Autodesk Fusion 360 part; units mm, degrees
(part 9 of 21)
  spline S252 degree 3 poles (-27.9507, 7.0582) (-27.9377, 7.0577) (-27.9248, 7.0598) (-27.9003, 7.0688) (-27.8891, 7.0756) (-27.8724, 7.0909) (-27.8662, 7.0984) (-27.8563, 7.115) (-27.8526, 7.124) (-27.8502, 7.1333) knots 0 0 0 0 0.003906 0.003906 0.007813 0.007813 0.010709 0.010709 0.013605 0.013605 0.013605 0.013605
  spline S253 degree 5 poles (-27.9507, 7.0582) (-27.9531, 7.0583) (-27.9637, 7.0587) (-27.9826, 7.0593) (-28.0098, 7.0601) (-28.0453, 7.061) (-28.0868, 7.0618) (-28.1283, 7.0622) (-28.1698, 7.0625) (-28.2114, 7.0625) (-28.253, 7.0622) (-28.2947, 7.0618) (-28.3364, 7.0611) (-28.3781, 7.0601) (-28.4199, 7.059) (-28.4617, 7.0576) (-28.5036, 7.0559) (-28.5454, 7.0541) (-28.5873, 7.0521) (-28.6293, 7.0498) (-28.6712, 7.0474) (-28.7132, 7.0447) (-28.7553, 7.0419) (-28.7973, 7.0388) (-28.8394, 7.0356) (-28.8815, 7.0321) (-28.9236, 7.0285) (-28.9658, 7.0247) (-29.0079, 7.0207) (-29.0501, 7.0165) (-29.0923, 7.0121) (-29.1346, 7.0075) (-29.1768, 7.0027) (-29.2191, 6.9978) (-29.2614, 6.9927) (-29.3037, 6.9874) (-29.3461, 6.982) (-29.3884, 6.9763) (-29.4308, 6.9705) (-29.4732, 6.9646) (-29.5156, 6.9584) (-29.558, 6.9521) (-29.6004, 6.9456) (-29.6429, 6.939) (-29.6854, 6.9321) (-29.7278, 6.9252) (-29.7703, 6.918) (-29.8128, 6.9107) (-29.8553, 6.9033) (-29.8979, 6.8956) (-29.9404, 6.8879) (-29.983, 6.8799) (-30.0255, 6.8718) (-30.0681, 6.8636) (-30.1107, 6.8552) (-30.1533, 6.8466) (-30.1873, 6.8396) (-30.2129, 6.8343) (-30.2299, 6.8308) (-30.2385, 6.829) knots 0.224488 0.224488 0.224488 0.224488 0.224488 0.224488 0.228571 0.242857 0.257143 0.271429 0.285714 0.3 0.314286 0.328571 0.342857 0.357143 0.371429 0.385714 0.4 0.414286 0.428571 0.442857 0.457143 0.471429 0.485714 0.5 0.514286 0.528571 0.542857 0.557143 0.571429 0.585714 0.6 0.614286 0.628571 0.642857 0.657143 0.671429 0.685714 0.7 0.714286 0.728571 0.742857 0.757143 0.771429 0.785714 0.8 0.814286 0.828571 0.842857 0.857143 0.871429 0.885714 0.9 0.914286 0.928571 0.942857 0.957143 0.971429 0.985714 1 1 1 1 1 1
  arc A157 (-30.2385, 6.829) -> (-30.4018, 6.0605) centre (0, 0) ccw
  spline S254 degree 5 poles (-30.4018, 6.0605) (-30.3948, 6.0554) (-30.3806, 6.0452) (-30.3594, 6.03) (-30.3311, 6.0097) (-30.2957, 5.9846) (-30.2602, 5.9596) (-30.2247, 5.9348) (-30.1891, 5.91) (-30.1535, 5.8855) (-30.1178, 5.8611) (-30.082, 5.8368) (-30.0462, 5.8127) (-30.0104, 5.7887) (-29.9744, 5.7649) (-29.9385, 5.7413) (-29.9025, 5.7178) (-29.8664, 5.6945) (-29.8303, 5.6713) (-29.7941, 5.6483) (-29.7578, 5.6254) (-29.7215, 5.6027) (-29.6852, 5.5802) (-29.6488, 5.5578) (-29.6123, 5.5356) (-29.5758, 5.5135) (-29.5393, 5.4917) (-29.5026, 5.47) (-29.466, 5.4484) (-29.4292, 5.4271) (-29.3925, 5.4059) (-29.3556, 5.3849) (-29.3187, 5.3641) (-29.2818, 5.3434) (-29.2448, 5.323) (-29.2077, 5.3027) (-29.1706, 5.2826) (-29.1334, 5.2627) (-29.0962, 5.243) (-29.0589, 5.2235) (-29.0216, 5.2042) (-28.9842, 5.1851) (-28.9467, 5.1662) (-28.9092, 5.1475) (-28.8716, 5.129) (-28.834, 5.1107) (-28.7963, 5.0927) (-28.7586, 5.0749) (-28.7208, 5.0572) (-28.6829, 5.0399) (-28.645, 5.0227) (-28.607, 5.0058) (-28.5689, 4.9891) (-28.5308, 4.9727) (-28.4926, 4.9565) (-28.4599, 4.9429) (-28.4347, 4.9326) (-28.4172, 4.9255) (-28.4073, 4.9215) (-28.4051, 4.9206) knots -1 -1 -1 -1 -1 -1 -0.985714 -0.971429 -0.957143 -0.942857 -0.928571 -0.914286 -0.9 -0.885714 -0.871429 -0.857143 -0.842857 -0.828571 -0.814286 -0.8 -0.785714 -0.771429 -0.757143 -0.742857 -0.728571 -0.714286 -0.7 -0.685714 -0.671429 -0.657143 -0.642857 -0.628571 -0.614286 -0.6 -0.585714 -0.571429 -0.557143 -0.542857 -0.528571 -0.514286 -0.5 -0.485714 -0.471429 -0.457143 -0.442857 -0.428571 -0.414286 -0.4 -0.385714 -0.371429 -0.357143 -0.342857 -0.328571 -0.314286 -0.3 -0.285714 -0.271429 -0.257143 -0.242857 -0.228571 -0.224488 -0.224488 -0.224488 -0.224488 -0.224488 -0.224488
  spline S255 degree 3 poles (-28.3438, 4.8111) (-28.3416, 4.8239) (-28.342, 4.8371) (-28.3477, 4.8625) (-28.353, 4.8745) (-28.366, 4.8931) (-28.3726, 4.9001) (-28.3878, 4.9121) (-28.3961, 4.917) (-28.4051, 4.9206) knots 0 0 0 0 0.003906 0.003906 0.007813 0.007813 0.010709 0.010709 0.013605 0.013605 0.013605 0.013605
  arc A158 (-28.3438, 4.8111) -> (-28.4432, 4.1831) centre (0, 0) ccw
  spline S256 degree 3 poles (-28.5354, 4.0979) (-28.5224, 4.0988) (-28.5097, 4.1022) (-28.4864, 4.1137) (-28.4759, 4.1216) (-28.4609, 4.1386) (-28.4556, 4.1467) (-28.4474, 4.1642) (-28.4447, 4.1735) (-28.4432, 4.1831) knots 0 0 0 0 0.003906 0.003906 0.007813 0.007813 0.010709 0.010709 0.013605 0.013605 0.013605 0.013605
  spline S257 degree 5 poles (-28.5354, 4.0979) (-28.5378, 4.0977) (-28.5484, 4.097) (-28.5672, 4.0957) (-28.5944, 4.0936) (-28.6298, 4.0908) (-28.6711, 4.0872) (-28.7124, 4.0833) (-28.7537, 4.0792) (-28.7951, 4.0749) (-28.8365, 4.0703) (-28.8778, 4.0655) (-28.9192, 4.0604) (-28.9607, 4.0551) (-29.0021, 4.0496) (-29.0435, 4.0438) (-29.085, 4.0379) (-29.1264, 4.0317) (-29.1679, 4.0253) (-29.2094, 4.0186) (-29.2508, 4.0118) (-29.2923, 4.0048) (-29.3338, 3.9976) (-29.3753, 3.9901) (-29.4168, 3.9825) (-29.4583, 3.9747) (-29.4998, 3.9667) (-29.5414, 3.9584) (-29.5829, 3.95) (-29.6244, 3.9415) (-29.6659, 3.9327) (-29.7075, 3.9237) (-29.749, 3.9146) (-29.7905, 3.9053) (-29.8321, 3.8958) (-29.8736, 3.8861) (-29.9151, 3.8762) (-29.9567, 3.8662) (-29.9982, 3.856) (-30.0397, 3.8456) (-30.0812, 3.8351) (-30.1228, 3.8244) (-30.1643, 3.8135) (-30.2058, 3.8024) (-30.2473, 3.7912) (-30.2889, 3.7798) (-30.3304, 3.7683) (-30.3719, 3.7566) (-30.4134, 3.7447) (-30.4549, 3.7327) (-30.4964, 3.7205) (-30.5379, 3.7082) (-30.5793, 3.6957) (-30.6208, 3.683) (-30.6623, 3.6702) (-30.7037, 3.6572) (-30.7369, 3.6467) (-30.7618, 3.6388) (-30.7784, 3.6335) (-30.7866, 3.6308) knots 0.224488 0.224488 0.224488 0.224488 0.224488 0.224488 0.228571 0.242857 0.257143 0.271429 0.285714 0.3 0.314286 0.328571 0.342857 0.357143 0.371429 0.385714 0.4 0.414286 0.428571 0.442857 0.457143 0.471429 0.485714 0.5 0.514286 0.528571 0.542857 0.557143 0.571429 0.585714 0.6 0.614286 0.628571 0.642857 0.657143 0.671429 0.685714 0.7 0.714286 0.728571 0.742857 0.757143 0.771429 0.785714 0.8 0.814286 0.828571 0.842857 0.857143 0.871429 0.885714 0.9 0.914286 0.928571 0.942857 0.957143 0.971429 0.985714 1 1 1 1 1 1
  arc A159 (-30.7866, 3.6308) -> (-30.8688, 2.8495) centre (0, 0) ccw
  spline S258 degree 5 poles (-30.8688, 2.8495) (-30.8612, 2.8451) (-30.8461, 2.8365) (-30.8234, 2.8235) (-30.7932, 2.8064) (-30.7553, 2.7851) (-30.7174, 2.7639) (-30.6795, 2.7429) (-30.6415, 2.722) (-30.6035, 2.7013) (-30.5654, 2.6808) (-30.5273, 2.6604) (-30.4892, 2.6402) (-30.451, 2.6201) (-30.4128, 2.6002) (-30.3746, 2.5804) (-30.3363, 2.5608) (-30.298, 2.5414) (-30.2596, 2.5221) (-30.2213, 2.503) (-30.1828, 2.484) (-30.1444, 2.4653) (-30.1059, 2.4466) (-30.0673, 2.4282) (-30.0287, 2.4099) (-29.9901, 2.3918) (-29.9515, 2.3739) (-29.9128, 2.3561) (-29.8741, 2.3386) (-29.8353, 2.3212) (-29.7965, 2.3039) (-29.7577, 2.2869) (-29.7188, 2.2701) (-29.6799, 2.2534) (-29.641, 2.2369) (-29.602, 2.2206) (-29.563, 2.2045) (-29.5239, 2.1886) (-29.4849, 2.1729) (-29.4457, 2.1574) (-29.4066, 2.1421) (-29.3674, 2.127) (-29.3282, 2.1122) (-29.2889, 2.0975) (-29.2496, 2.083) (-29.2103, 2.0688) (-29.1709, 2.0548) (-29.1315, 2.041) (-29.0921, 2.0274) (-29.0526, 2.0141) (-29.0131, 2.001) (-28.9735, 1.9881) (-28.9339, 1.9755) (-28.8943, 1.9632) (-28.8546, 1.9511) (-28.8206, 1.9409) (-28.7945, 1.9333) (-28.7763, 1.9281) (-28.7661, 1.9252) (-28.7638, 1.9245) knots -1 -1 -1 -1 -1 -1 -0.985714 -0.971429 -0.957143 -0.942857 -0.928571 -0.914286 -0.9 -0.885714 -0.871429 -0.857143 -0.842857 -0.828571 -0.814286 -0.8 -0.785714 -0.771429 -0.757143 -0.742857 -0.728571 -0.714286 -0.7 -0.685714 -0.671429 -0.657143 -0.642857 -0.628571 -0.614286 -0.6 -0.585714 -0.571429 -0.557143 -0.542857 -0.528571 -0.514286 -0.5 -0.485714 -0.471429 -0.457143 -0.442857 -0.428571 -0.414286 -0.4 -0.385714 -0.371429 -0.357143 -0.342857 -0.328571 -0.314286 -0.3 -0.285714 -0.271429 -0.257143 -0.242857 -0.228571 -0.224488 -0.224488 -0.224488 -0.224488 -0.224488 -0.224488
  spline S259 degree 3 poles (-28.6914, 1.822) (-28.6906, 1.835) (-28.6923, 1.848) (-28.7006, 1.8727) (-28.7072, 1.8841) (-28.7221, 1.9012) (-28.7294, 1.9075) (-28.7457, 1.9179) (-28.7546, 1.9219) (-28.7638, 1.9245) knots 0 0 0 0 0.003906 0.003906 0.007813 0.007813 0.010709 0.010709 0.013605 0.013605 0.013605 0.013605
  line L20 (0, 31) -> (0, 3.7492)
  line L21 (2.2037, 3.0332) -> (18.2213, 25.0795)
  circle A160 centre (0, 0) radius 7.5
  circle A161 centre (0, 0) radius 27.5
  dimension "d19" = 36
  dimension "d20" = 15
  dimension "d21" = 55
  constraint vertical L20
  constraint coincident A1.centre L20
  constraint coincident A1.centre L21
  constraint coincident A9 L20.end
  constraint coincident A13 L21.start
  constraint coincident A131 L20.start
  constraint coincident A119 L21.end
  constraint coincident A1.centre A3.centre
  constraint concentric A1 A161
  measures "d19" angle of L20 L21
  measures "d20" diameter of A160
  measures "d21" diameter of A161
extrude "Estrusione4" cut sketch "Schizzo1 (3)" against normal blind 1 contours L20 L21 A160 A161 picked at (8.9949, 18.7465) bodies 1 in component "Spur Gear (60 teeth)"
pattern_circular "Serie C2" count 5 over 360 about axis through (0, 0, 0) along (0, 0, 1) of "Estrusione4" in component "Spur Gear (60 teeth)"
extrude "Estrusione5" cut 1 faces at (-3.6482, -2.3787, 8) along direction (0, 0, -1) blind 1.6 on bodies 1 bodies 1 in component "Spur Gear (60 teeth)"
sketch "Schizzo2 (3)" plane through (0, 0, 2) normal (0, 0, 1) x (-1, 0, 0)
  line L0 (7.1329, -2.3176) -> (26.1541, -8.498)
  arc A0 (26.1541, -8.498) -> (26.1541, 8.498) centre (0, 0) ccw
  line L1 (26.1541, 8.498) -> (7.1329, 2.3176)
  arc A1 (7.1329, -2.3176) -> (7.1329, 2.3176) centre (0, 0) ccw
  line L2 (24.4009, 8.0452) -> (-1.5991, 8.0452) construction
  line L3 (-1.5991, 8.0452) -> (-1.5991, -2.9548) construction
  line L4 (-1.5991, -2.9548) -> (24.4009, -2.9548) construction
  line L5 (24.4009, -2.9548) -> (24.4009, 8.0452) construction
  dimension "d28" = 5
  text T0 "60s" font "Arial" height 5 bold align left top in box 26 x 11 at (24.4009, 8.0452) x (-1, 0) y (0, -1) spacing 1 kerned
extrude "Estrusione6" add sketch "Schizzo2 (3)" along normal blind 1 text T0 bodies 1 in component "Spur Gear (60 teeth)"
component "Spur Gear (60 teeth)" placed x (1, 0, 0) y (0, 1, 0) z (0, 0, 1) at (0, 0, 0)
component "Spur Gear (10 teeth)" placed x (1, 0, 0) y (0, 1, 0) z (0, 0, 1) at (0, 0, 0)
equation "d19 = ( 360 / 10 ) * 1 deg"

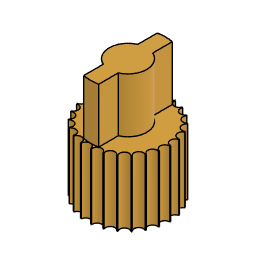
design "2 pomello lancetta secondi"
Autodesk Fusion 360 part; units mm, degrees
sketch "Schizzo1" plane through (0, 0, 0) normal (0, 0, 1) x (1, 0, 0)
  line L0 (0, -45) -> (5, 0)
  line L1 (5, 0) -> (0, 15)
  line L2 (0, 15) -> (-5, 0)
  line L3 (-5, 0) -> (0, -45)
  line L4 (0, -45) -> (0, 15) construction
  line L5 (5, 0) -> (-5, 0) construction
  line L6 (-1, 15) -> (1, 15)
  line L7 (1, 15) -> (1, -45)
  line L8 (1, -45) -> (-1, -45)
  line L9 (-1, -45) -> (-1, 15)
  circle A0 centre (0, 0) radius 5
  dimension "d1" = 45
  dimension "d2" = 15
  dimension "d3" = 5
  dimension "d12" = 1
  dimension "d13" = 1
  constraint vertical L4
  constraint perpendicular L4 L5
  constraint midpoint A0.centre L5
  constraint equal L0 L3
  constraint equal L1 L2
  constraint horizontal L6
  constraint vertical L7
  constraint horizontal L8
  constraint vertical L9
  constraint coincident A0.centre origin
  constraint coincident L0.end A0
  constraint midpoint L0.start L8
  constraint midpoint L1.end L6
  measures "d1" vertical distance of L0.start L0.end
  measures "d2" vertical distance of L0.end L1.end
  measures "d3" horizontal distance of L0.start L0.end
  measures "d12" distance of A0.centre L9
  measures "d13" distance of A0.centre L7
extrude "Estrusione1" add sketch "Schizzo1" along normal blind 2 contours L0 L3 L7 L9 A0 | L3 L8 L9 | L0 L7 L8 | L0 L1 L7 A0 | L0 A0 | L7 L9 A0 | L3 A0 | L2 L3 L9 A0 | L1 A0 | L1 L2 L7 L9 A0 | L2 A0 | L1 L6 L7 | L2 L6 L9
sketch "Schizzo2" plane through (0, 0, 2) normal (0, 0, 1) x (-1, 0, 0)
  circle A0 centre (0, 0) radius 2
  circle A1 centre (0, 0) radius 4
  line L0 (-0.8, 24) -> (0.8, 24)
  line L1 (0.8, 24) -> (0.8, -21)
  line L2 (0.8, -21) -> (-0.8, -21)
  line L3 (-0.8, -21) -> (-0.8, 24)
  arc A2 (-1, 4.899) -> (-1, -4.899) centre (0, 0) ccw
  line L4 (-1, -4.899) -> (-1, -15)
  line L5 (-1, -15) -> (1, -15)
  line L6 (1, -15) -> (1, -4.899)
  arc A3 (1, -4.899) -> (1, 4.899) centre (0, 0) ccw
  line L7 (1, 4.899) -> (1, 45)
  line L8 (-1, 45) -> (-1, 4.899)
  line L9 (1, 45) -> (-1, 45)
  dimension "d6" = 4
  dimension "d7" = 8
  dimension "d8" = 0.8
  dimension "d9" = 0.8
  constraint coincident A0.centre A1.centre
  constraint horizontal L0
  constraint vertical L1
  constraint horizontal L2
  constraint vertical L3
  measures "d6" diameter of A0
  measures "d7" diameter of A1
  measures "d8" distance of A0.centre L3
  measures "d9" distance of A0.centre L1
extrude "Estrusione2" add sketch "Schizzo2" along normal blind 3.8 contours A0 L1 | A0 L1 L3 | A0 A1 L1 L3 | A0 A1 L1 L3 | A0 L3
extrude "Estrusione3" add 1 faces at (0.3333, -45, 0.6667) along direction (0, -1, 0) blind 10
sketch "Schizzo3" plane through (0, 0, 0) normal (0, 0, -1) x (1, 0, 0)
  line L0 (1, 4.899) -> (1, 55)
  line L1 (1, 55) -> (-1, 55)
  line L2 (-1, 55) -> (-1, 4.899)
  arc A0 (-1, 4.899) -> (-1, -4.899) centre (0, 0) ccw
  line L3 (-1, -4.899) -> (-1, -15)
  line L4 (-1, -15) -> (1, -15)
  line L5 (1, -15) -> (1, -4.899)
  arc A1 (1, -4.899) -> (1, 4.899) centre (0, 0) ccw
  circle A2 centre (0, 0) radius 6
  dimension "d16" = 12
  constraint concentric A0 A2
  measures "d16" diameter of A2
extrude "Estrusione4" add sketch "Schizzo3" against normal up to surface (2 mm away) contours L0 L5 A1 A2 | L2 A0 L3 A2
sketch "Schizzo4" plane through (0, 0, 0) normal (0, 0, -1) x (1, 0, 0)
  line L0 (1, 5.9161) -> (1, 55)
  line L1 (1, 55) -> (-1, 55)
  line L2 (-1, 55) -> (-1, 5.9161)
  arc A0 (-1, 5.9161) -> (-1, -5.9161) centre (0, 0) ccw
  line L3 (-1, -5.9161) -> (-1, -15)
  line L4 (-1, -15) -> (1, -15)
  line L5 (1, -15) -> (1, -5.9161)
  arc A1 (1, -5.9161) -> (1, 5.9161) centre (0, 0) ccw
  circle A2 centre (0, 0) radius 4.5
  circle A3 centre (0, 4.5) radius 0.5
  circle A4 centre (-1.0769, 4.3692) radius 0.5
  circle A5 centre (-2.0913, 3.9846) radius 0.5
  circle A6 centre (-2.9841, 3.3683) radius 0.5
  circle A7 centre (-3.7034, 2.5563) radius 0.5
  circle A8 centre (-4.2076, 1.5957) radius 0.5
  circle A9 centre (-4.4672, 0.5424) radius 0.5
  circle A10 centre (-4.4672, -0.5424) radius 0.5
  circle A11 centre (-4.2076, -1.5957) radius 0.5
  circle A12 centre (-3.7034, -2.5563) radius 0.5
  circle A13 centre (-2.9841, -3.3683) radius 0.5
  circle A14 centre (-2.0913, -3.9846) radius 0.5
  circle A15 centre (-1.0769, -4.3692) radius 0.5
  circle A16 centre (0, -4.5) radius 0.5
  circle A17 centre (1.0769, -4.3692) radius 0.5
  circle A18 centre (2.0913, -3.9846) radius 0.5
  circle A19 centre (2.9841, -3.3683) radius 0.5
  circle A20 centre (3.7034, -2.5563) radius 0.5
  circle A21 centre (4.2076, -1.5957) radius 0.5
  circle A22 centre (4.4672, -0.5424) radius 0.5
  circle A23 centre (4.4672, 0.5424) radius 0.5
  circle A24 centre (4.2076, 1.5957) radius 0.5
  circle A25 centre (3.7034, 2.5563) radius 0.5
  circle A26 centre (2.9841, 3.3683) radius 0.5
  circle A27 centre (2.0913, 3.9846) radius 0.5
  circle A28 centre (1.0769, 4.3692) radius 0.5
  dimension "d19" = 9
  dimension "d20" = 1
  dimension "d22" = 360
  constraint coincident A0.centre A1.centre
  constraint coincident A2 A3.centre
  measures "d19" diameter of A2
  measures "d20" diameter of A3
extrude "Estrusione5" add sketch "Schizzo4" along normal blind 7 contours A2 A3 A4 A5 A6 A7 A8 A9 A10 A11 A12 A13 A14 A15 A16 A17 A18 A19 A20 A21 A22 A23 A24 A25 A26 A27 A28
sketch "Schizzo5" plane through (0, 0, 2) normal (0, 0, 1) x (-1, 0, 0)
  line L0 (-0.8, 1.833) -> (-0.8, 3.9192)
  arc A0 (0.8, 3.9192) -> (-0.8, 3.9192) centre (0, 0) ccw
  line L1 (0.8, 3.9192) -> (0.8, 1.833)
  arc A1 (0.8, -1.833) -> (0.8, 1.833) centre (0, 0) ccw
  line L2 (0.8, -1.833) -> (0.8, -3.9192)
  arc A2 (-0.8, -3.9192) -> (0.8, -3.9192) centre (0, 0) ccw
  line L3 (-0.8, -3.9192) -> (-0.8, -1.833)
  arc A3 (-0.8, 1.833) -> (-0.8, -1.833) centre (0, 0) ccw
  line L4 (-1, -5.9161) -> (-1, -15)
  line L5 (-1, -15) -> (1, -15)
  line L6 (1, -15) -> (1, -5.9161)
  arc A4 (1, -5.9161) -> (1, 5.9161) centre (0, 0) ccw
  line L7 (1, 5.9161) -> (1, 55)
  line L8 (1, 55) -> (-1, 55)
  line L9 (-1, 55) -> (-1, 5.9161)
  arc A5 (-1, 5.9161) -> (-1, -5.9161) centre (0, 0) ccw
extrude "Estrusione6" cut sketch "Schizzo5" against normal up to surface (2 mm away)
sketch "Schizzo6" plane through (0, 0, -7) normal (0, 0, -1) x (1, 0, 0)
  arc A0 (2.592, 3.6786) -> (2.5204, 3.728) centre (0, 0) ccw
  arc A1 (1.6363, 4.192) -> (2.5204, 3.728) centre (2.0913, 3.9846) ccw
  arc A2 (1.6363, 4.192) -> (1.555, 4.2228) centre (0, 0) ccw
  arc A3 (0.5856, 4.4617) -> (1.555, 4.2228) centre (1.0769, 4.3692) ccw
  arc A4 (0.5856, 4.4617) -> (0.4992, 4.4722) centre (0, 0) ccw
  arc A5 (-0.4992, 4.4722) -> (0.4992, 4.4722) centre (0, 4.5) ccw
  arc A6 (-0.4992, 4.4722) -> (-0.5856, 4.4617) centre (0, 0) ccw
  arc A7 (-1.555, 4.2228) -> (-0.5856, 4.4617) centre (-1.0769, 4.3692) ccw
  arc A8 (-1.555, 4.2228) -> (-1.6363, 4.192) centre (0, 0) ccw
  arc A9 (-2.5204, 3.728) -> (-1.6363, 4.192) centre (-2.0913, 3.9846) ccw
  arc A10 (-2.5204, 3.728) -> (-2.592, 3.6786) centre (0, 0) ccw
  arc A11 (-3.3393, 3.0165) -> (-2.592, 3.6786) centre (-2.9841, 3.3683) ccw
  arc A12 (-3.3393, 3.0165) -> (-3.397, 2.9514) centre (0, 0) ccw
  arc A13 (-3.9642, 2.1297) -> (-3.397, 2.9514) centre (-3.7034, 2.5563) ccw
  arc A14 (-3.9642, 2.1297) -> (-4.0046, 2.0527) centre (0, 0) ccw
  arc A15 (-4.3586, 1.1191) -> (-4.0046, 2.0527) centre (-4.2076, 1.5957) ccw
  arc A16 (-4.3586, 1.1191) -> (-4.3794, 1.0347) centre (0, 0) ccw
  arc A17 (-4.4998, 0.0435) -> (-4.3794, 1.0347) centre (-4.4672, 0.5424) ccw
  arc A18 (-4.4998, 0.0435) -> (-4.4998, -0.0435) centre (0, 0) ccw
  arc A19 (-4.3794, -1.0347) -> (-4.4998, -0.0435) centre (-4.4672, -0.5424) ccw
  arc A20 (-4.3794, -1.0347) -> (-4.3586, -1.1191) centre (0, 0) ccw
  arc A21 (-4.0046, -2.0527) -> (-4.3586, -1.1191) centre (-4.2076, -1.5957) ccw
  arc A22 (-4.0046, -2.0527) -> (-3.9642, -2.1297) centre (0, 0) ccw
  arc A23 (-3.397, -2.9514) -> (-3.9642, -2.1297) centre (-3.7034, -2.5563) ccw
  arc A24 (-3.397, -2.9514) -> (-3.3393, -3.0165) centre (0, 0) ccw
  arc A25 (-2.592, -3.6786) -> (-3.3393, -3.0165) centre (-2.9841, -3.3683) ccw
  arc A26 (-2.592, -3.6786) -> (-2.5204, -3.728) centre (0, 0) ccw
  arc A27 (-1.6363, -4.192) -> (-2.5204, -3.728) centre (-2.0913, -3.9846) ccw
  arc A28 (-1.6363, -4.192) -> (-1.555, -4.2228) centre (0, 0) ccw
  arc A29 (-0.5856, -4.4617) -> (-1.555, -4.2228) centre (-1.0769, -4.3692) ccw
  arc A30 (-0.5856, -4.4617) -> (-0.4992, -4.4722) centre (0, 0) ccw
  arc A31 (0.4992, -4.4722) -> (-0.4992, -4.4722) centre (0, -4.5) ccw
  arc A32 (0.4992, -4.4722) -> (0.5856, -4.4617) centre (0, 0) ccw
  arc A33 (1.555, -4.2228) -> (0.5856, -4.4617) centre (1.0769, -4.3692) ccw
  arc A34 (1.555, -4.2228) -> (1.6363, -4.192) centre (0, 0) ccw
  arc A35 (2.5204, -3.728) -> (1.6363, -4.192) centre (2.0913, -3.9846) ccw
  arc A36 (2.5204, -3.728) -> (2.592, -3.6786) centre (0, 0) ccw
  arc A37 (3.3393, -3.0165) -> (2.592, -3.6786) centre (2.9841, -3.3683) ccw
  arc A38 (3.3393, -3.0165) -> (3.397, -2.9514) centre (0, 0) ccw
  arc A39 (3.9642, -2.1297) -> (3.397, -2.9514) centre (3.7034, -2.5563) ccw
  arc A40 (3.9642, -2.1297) -> (4.0046, -2.0527) centre (0, 0) ccw
  arc A41 (4.3586, -1.1191) -> (4.0046, -2.0527) centre (4.2076, -1.5957) ccw
  arc A42 (4.3586, -1.1191) -> (4.3794, -1.0347) centre (0, 0) ccw
  arc A43 (4.4998, -0.0435) -> (4.3794, -1.0347) centre (4.4672, -0.5424) ccw
  arc A44 (4.4998, -0.0435) -> (4.4998, 0.0435) centre (0, 0) ccw
  arc A45 (4.3794, 1.0347) -> (4.4998, 0.0435) centre (4.4672, 0.5424) ccw
  arc A46 (4.3794, 1.0347) -> (4.3586, 1.1191) centre (0, 0) ccw
  arc A47 (4.0046, 2.0527) -> (4.3586, 1.1191) centre (4.2076, 1.5957) ccw
  arc A48 (4.0046, 2.0527) -> (3.9642, 2.1297) centre (0, 0) ccw
  arc A49 (3.397, 2.9514) -> (3.9642, 2.1297) centre (3.7034, 2.5563) ccw
  arc A50 (3.397, 2.9514) -> (3.3393, 3.0165) centre (0, 0) ccw
  arc A51 (2.592, 3.6786) -> (3.3393, 3.0165) centre (2.9841, 3.3683) ccw
  line L0 (-1.5, 8) -> (1.5, 8)
  line L1 (1.5, 8) -> (1.5, -40)
  line L2 (1.5, -40) -> (-1.5, -40)
  line L3 (-1.5, -40) -> (-1.5, 8)
  dimension "d27" = 8
  dimension "d28" = 40
  dimension "d29" = 3
  dimension "d30" = 1.5
  constraint horizontal L0
  constraint vertical L1
  constraint horizontal L2
  constraint vertical L3
  measures "d27" distance of A0.centre L0
  measures "d28" distance of A0.centre L2
  measures "d29" distance of L0.start L0.end
  measures "d30" distance of A0.centre L3
extrude "Estrusione7" [rolled back] along distance -9 taper angle 0
sketch "Schizzo7" plane through (0, 0, 0) normal (0, 0, 1) x (-1, 0, 0)
  line L0 (1.5, -1.3229) -> (1.5, -4.1028)
  arc A0 (1.555, -4.2228) -> (1.5, -4.1028) centre (1.0769, -4.3692) ccw
  arc A1 (1.555, -4.2228) -> (1.6363, -4.192) centre (0, 0) ccw
  arc A2 (2.5204, -3.728) -> (1.6363, -4.192) centre (2.0913, -3.9846) ccw
  arc A3 (2.5204, -3.728) -> (2.592, -3.6786) centre (0, 0) ccw
  arc A4 (3.3393, -3.0165) -> (2.592, -3.6786) centre (2.9841, -3.3683) ccw
  arc A5 (3.3393, -3.0165) -> (3.397, -2.9514) centre (0, 0) ccw
  arc A6 (3.9642, -2.1297) -> (3.397, -2.9514) centre (3.7034, -2.5563) ccw
  arc A7 (3.9642, -2.1297) -> (4.0046, -2.0527) centre (0, 0) ccw
  arc A8 (4.3586, -1.1191) -> (4.0046, -2.0527) centre (4.2076, -1.5957) ccw
  arc A9 (4.3586, -1.1191) -> (4.3794, -1.0347) centre (0, 0) ccw
  arc A10 (4.4998, -0.0435) -> (4.3794, -1.0347) centre (4.4672, -0.5424) ccw
  arc A11 (4.4998, -0.0435) -> (4.4998, 0.0435) centre (0, 0) ccw
  arc A12 (4.3794, 1.0347) -> (4.4998, 0.0435) centre (4.4672, 0.5424) ccw
  arc A13 (4.3794, 1.0347) -> (4.3586, 1.1191) centre (0, 0) ccw
  arc A14 (4.0046, 2.0527) -> (4.3586, 1.1191) centre (4.2076, 1.5957) ccw
  arc A15 (4.0046, 2.0527) -> (3.9642, 2.1297) centre (0, 0) ccw
  arc A16 (3.397, 2.9514) -> (3.9642, 2.1297) centre (3.7034, 2.5563) ccw
  arc A17 (3.397, 2.9514) -> (3.3393, 3.0165) centre (0, 0) ccw
  arc A18 (2.592, 3.6786) -> (3.3393, 3.0165) centre (2.9841, 3.3683) ccw
  arc A19 (2.592, 3.6786) -> (2.5204, 3.728) centre (0, 0) ccw
  arc A20 (1.6363, 4.192) -> (2.5204, 3.728) centre (2.0913, 3.9846) ccw
  arc A21 (1.6363, 4.192) -> (1.555, 4.2228) centre (0, 0) ccw
  arc A22 (1.5, 4.1028) -> (1.555, 4.2228) centre (1.0769, 4.3692) ccw
  line L1 (1.5, 4.1028) -> (1.5, 1.3229)
  arc A23 (1.5, -1.3229) -> (1.5, 1.3229) centre (0, 0) ccw
  circle A24 centre (0, 0) radius 5
  constraint coincident A1.centre A3.centre
extrude "Estrusione8" [rolled back] side1offset 0 taper angle 0

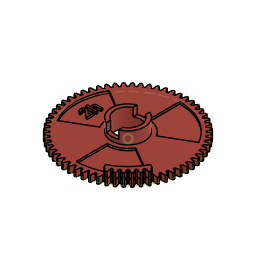
design "7 ore"
description: Spur Gear; Module: 0.930000; Num Teeth: 60; Pressure Angle: 20.000000; Backlash: 0.00 mm
Autodesk Fusion 360 part; units mm, degrees
sketch "Schizzo1" plane through (0, 0, 0) normal (0, 0, 1) x (1, 0, 0) in component "Spur Gear (60 teeth) (1)"
  circle A0 centre (0, 0) radius 26.7332
  circle A1 centre (0, 0) radius 4.1
extrude "Estrusione1" add sketch "Schizzo1" along normal blind 6 in component "Spur Gear (60 teeth) (1)"
sketch "Schizzo2" plane through (0, 0, 0) normal (0, 0, 1) x (1, 0, 0) in component "Spur Gear (60 teeth) (1)"
  spline S0 degree 5 poles (26.1953, -1.0768) (26.2029, -1.0768) (26.218, -1.0767) (26.2407, -1.0765) (26.271, -1.0757) (26.3089, -1.0742) (26.3468, -1.0722) (26.3847, -1.0696) (26.4226, -1.0664) (26.4605, -1.0628) (26.4984, -1.0587) (26.5363, -1.0542) (26.5742, -1.0494) (26.6121, -1.0443) (26.65, -1.0388) (26.6879, -1.0332) (26.7258, -1.0272) (26.7637, -1.0209) (26.8015, -1.0144) (26.8394, -1.0076) (26.8773, -1.0005) (26.9151, -0.9932) (26.953, -0.9856) (26.9908, -0.9778) (27.0286, -0.9697) (27.0664, -0.9615) (27.1042, -0.953) (27.142, -0.9443) (27.1798, -0.9354) (27.2176, -0.9262) (27.2553, -0.9169) (27.2931, -0.9073) (27.3308, -0.8976) (27.3686, -0.8876) (27.4063, -0.8775) (27.444, -0.8671) (27.4817, -0.8566) (27.5193, -0.8459) (27.557, -0.835) (27.5946, -0.8239) (27.6323, -0.8126) (27.6699, -0.8011) (27.7075, -0.7895) (27.7451, -0.7777) (27.7827, -0.7657) (27.8202, -0.7536) (27.8578, -0.7412) (27.8953, -0.7288) (27.9328, -0.7161) (27.9703, -0.7033) (28.0078, -0.6903) (28.0452, -0.6771) (28.0827, -0.6638) (28.1201, -0.6503) (28.1575, -0.6367) (28.1949, -0.6229) (28.2323, -0.609) (28.2697, -0.5949) (28.307, -0.5806) (28.3443, -0.5662) (28.3816, -0.5516) (28.4189, -0.5369) (28.4562, -0.522) (28.4934, -0.507) (28.5306, -0.4919) (28.5678, -0.4766) (28.605, -0.4611) (28.6422, -0.4455) (28.6793, -0.4298) (28.7164, -0.4139) (28.7535, -0.3978) (28.7832, -0.3849) (28.8055, -0.3751) (28.8203, -0.3686) (28.8277, -0.3653) knots 0 0 0 0 0 0 0.01428571 0.02857143 0.04285714 0.05714286 0.07142857 0.08571429 0.1 0.11428571 0.12857143 0.14285714 0.15714286 0.17142857 0.18571429 0.2 0.21428571 0.22857143 0.24285714 0.25714286 0.27142857 0.28571429 0.3 0.31428571 0.32857143 0.34285714 0.35714286 0.37142857 0.38571429 0.4 0.41428571 0.42857143 0.44285714 0.45714286 0.47142857 0.48571429 0.5 0.51428571 0.52857143 0.54285714 0.55714286 0.57142857 0.58571429 0.6 0.61428571 0.62857143 0.64285714 0.65714286 0.67142857 0.68571429 0.7 0.71428571 0.72857143 0.74285714 0.75714286 0.77142857 0.78571429 0.8 0.81428571 0.82857143 0.84285714 0.85714286 0.87142857 0.88571429 0.9 0.91428571 0.92857143 0.94285714 0.95714286 0.97142857 0.98571429 1 1 1 1 1 1
  spline S1 degree 5 poles (26.1953, 1.0768) (26.2029, 1.0768) (26.218, 1.0767) (26.2407, 1.0765) (26.271, 1.0757) (26.3089, 1.0742) (26.3468, 1.0722) (26.3847, 1.0696) (26.4226, 1.0664) (26.4605, 1.0628) (26.4984, 1.0587) (26.5363, 1.0542) (26.5742, 1.0494) (26.6121, 1.0443) (26.65, 1.0388) (26.6879, 1.0332) (26.7258, 1.0272) (26.7637, 1.0209) (26.8015, 1.0144) (26.8394, 1.0076) (26.8773, 1.0005) (26.9151, 0.9932) (26.953, 0.9856) (26.9908, 0.9778) (27.0286, 0.9697) (27.0664, 0.9615) (27.1042, 0.953) (27.142, 0.9443) (27.1798, 0.9354) (27.2176, 0.9262) (27.2553, 0.9169) (27.2931, 0.9073) (27.3308, 0.8976) (27.3686, 0.8876) (27.4063, 0.8775) (27.444, 0.8671) (27.4817, 0.8566) (27.5193, 0.8459) (27.557, 0.835) (27.5946, 0.8239) (27.6323, 0.8126) (27.6699, 0.8011) (27.7075, 0.7895) (27.7451, 0.7777) (27.7827, 0.7657) (27.8202, 0.7536) (27.8578, 0.7412) (27.8953, 0.7288) (27.9328, 0.7161) (27.9703, 0.7033) (28.0078, 0.6903) (28.0452, 0.6771) (28.0827, 0.6638) (28.1201, 0.6503) (28.1575, 0.6367) (28.1949, 0.6229) (28.2323, 0.609) (28.2697, 0.5949) (28.307, 0.5806) (28.3443, 0.5662) (28.3816, 0.5516) (28.4189, 0.5369) (28.4562, 0.522) (28.4934, 0.507) (28.5306, 0.4919) (28.5678, 0.4766) (28.605, 0.4611) (28.6422, 0.4455) (28.6793, 0.4298) (28.7164, 0.4139) (28.7535, 0.3978) (28.7832, 0.3849) (28.8055, 0.3751) (28.8203, 0.3686) (28.8277, 0.3653) knots 0 0 0 0 0 0 0.01428571 0.02857143 0.04285714 0.05714286 0.07142857 0.08571429 0.1 0.11428571 0.12857143 0.14285714 0.15714286 0.17142857 0.18571429 0.2 0.21428571 0.22857143 0.24285714 0.25714286 0.27142857 0.28571429 0.3 0.31428571 0.32857143 0.34285714 0.35714286 0.37142857 0.38571429 0.4 0.41428571 0.42857143 0.44285714 0.45714286 0.47142857 0.48571429 0.5 0.51428571 0.52857143 0.54285714 0.55714286 0.57142857 0.58571429 0.6 0.61428571 0.62857143 0.64285714 0.65714286 0.67142857 0.68571429 0.7 0.71428571 0.72857143 0.74285714 0.75714286 0.77142857 0.78571429 0.8 0.81428571 0.82857143 0.84285714 0.85714286 0.87142857 0.88571429 0.9 0.91428571 0.92857143 0.94285714 0.95714286 0.97142857 0.98571429 1 1 1 1 1 1
  arc A0 (28.8277, -0.3653) -> (28.8277, 0.3653) centre (0, 0) ccw
  line L0 (26.1953, 1.0768) -> (26.1953, -1.0768)
  point P0 (26.3824, -1.0696)
  point P1 (26.5699, -1.0499)
  point P2 (26.7578, -1.0218)
  point P3 (26.9458, -0.987)
  point P4 (27.134, -0.9461)
  point P5 (27.3223, -0.8997)
  point P6 (27.5106, -0.8483)
  point P7 (27.699, -0.7921)
  point P8 (27.8873, -0.7314)
  point P9 (28.0756, -0.6663)
  point P10 (28.2639, -0.597)
  point P11 (28.452, -0.5237)
  point P12 (28.6399, -0.4464)
  point P13 (26.3824, 1.0696)
  point P14 (26.5699, 1.0499)
  point P15 (26.7578, 1.0218)
  point P16 (26.9458, 0.987)
  point P17 (27.134, 0.9461)
  point P18 (27.3223, 0.8997)
  point P19 (27.5106, 0.8483)
  point P20 (27.699, 0.7921)
  point P21 (27.8873, 0.7314)
  point P22 (28.0756, 0.6663)
  point P23 (28.2639, 0.597)
  point P24 (28.452, 0.5237)
  point P25 (28.6399, 0.4464)
extrude "Estrusione2" add sketch "Schizzo2" along normal blind 6 in component "Spur Gear (60 teeth) (1)"
fillet "Raccordo1" radius 0.1 2 edges at (26.7134, 1.0291, 3) (26.7134, -1.0291, 3) in component "Spur Gear (60 teeth) (1)"
pattern_circular "Serie C1" count 60 over 360 about axis through (0, 0, 0) along (0, 0, 1) of "Estrusione2", "Raccordo1" in component "Spur Gear (60 teeth) (1)"
sketch "Schizzo3" plane through (0, 0, 0) normal (0, 0, 1) x (1, 0, 0) in component "Spur Gear (60 teeth) (1)"
  circle A0 centre (0, 0) radius 27.9 construction
extrude "Estrusione3" cut 1 faces at (19.1734, 0, 6) along direction (0, 0, -1) blind 3 in component "Spur Gear (60 teeth) (1)"
sketch "Schizzo3 (2)" plane through (0, 0, 3) normal (0, 0, 1) x (-1, 0, 0)
  arc A0 (-26.6799, 1.6879) -> (-26.7101, 1.1102) centre (0, 0) ccw
  spline S0 degree 3 poles (-26.7929, 1.0158) (-26.7834, 1.0175) (-26.7741, 1.0205) (-26.7569, 1.0291) (-26.7489, 1.0346) (-26.7323, 1.0501) (-26.7246, 1.0607) (-26.7138, 1.0844) (-26.7107, 1.0972) (-26.7101, 1.1102) knots -0.013599 -0.013599 -0.013599 -0.013599 -0.010706 -0.010706 -0.007813 -0.007813 -0.003906 -0.003906 0 0 0 0
  spline S1 degree 3 poles (-28.8277, 0.3653) (-28.4872, 0.5159) (-28.1325, 0.6536) (-27.4612, 0.8687) (-27.1231, 0.9582) (-26.7929, 1.0158) knots -0.220678 -0.220678 -0.220678 -0.220678 -0.107909 -0.107909 -0.008028 -0.008028 -0.008028 -0.008028
  arc A1 (-28.8277, 0.3653) -> (-28.8277, -0.3653) centre (0, 0) ccw
  spline S2 degree 3 poles (-26.7929, -1.0158) (-27.1231, -0.9582) (-27.4612, -0.8687) (-28.1325, -0.6536) (-28.4872, -0.5159) (-28.8277, -0.3653) knots -0.210627 -0.210627 -0.210627 -0.210627 -0.111696 -0.111696 0 0 0 0
  spline S3 degree 3 poles (-26.7101, -1.1102) (-26.7105, -1.1006) (-26.7123, -1.091) (-26.7186, -1.0728) (-26.723, -1.0642) (-26.7362, -1.0457) (-26.7457, -1.0367) (-26.7678, -1.0228) (-26.78, -1.0181) (-26.7929, -1.0158) knots -0.013599 -0.013599 -0.013599 -0.013599 -0.010706 -0.010706 -0.007813 -0.007813 -0.003906 -0.003906 0 0 0 0
  arc A2 (-26.7101, -1.1102) -> (-26.6799, -1.6879) centre (0, 0) ccw
  spline S4 degree 3 poles (-26.7523, -1.7903) (-26.743, -1.7877) (-26.7341, -1.7837) (-26.7179, -1.7734) (-26.7105, -1.7671) (-26.6957, -1.75) (-26.6891, -1.7386) (-26.6808, -1.7139) (-26.679, -1.7008) (-26.6799, -1.6879) knots -0.013599 -0.013599 -0.013599 -0.013599 -0.010706 -0.010706 -0.007813 -0.007813 -0.003906 -0.003906 0 0 0 0
  spline S5 degree 3 poles (-28.708, -2.65) (-28.385, -2.4646) (-28.0467, -2.2907) (-27.4015, -2.0065) (-27.0747, -1.8822) (-26.7523, -1.7903) knots -0.220678 -0.220678 -0.220678 -0.220678 -0.107909 -0.107909 -0.008028 -0.008028 -0.008028 -0.008028
  arc A3 (-28.708, -2.65) -> (-28.6316, -3.3766) centre (0, 0) ccw
  spline S6 degree 3 poles (-26.5399, -3.8109) (-26.8744, -3.7881) (-27.2199, -3.7344) (-27.9101, -3.5906) (-28.2772, -3.4908) (-28.6316, -3.3766) knots -0.210627 -0.210627 -0.210627 -0.210627 -0.111696 -0.111696 0 0 0 0
  spline S7 degree 3 poles (-26.4478, -3.8961) (-26.4492, -3.8865) (-26.452, -3.8773) (-26.4601, -3.8598) (-26.4654, -3.8517) (-26.4804, -3.8347) (-26.4908, -3.8267) (-26.5142, -3.8152) (-26.5269, -3.8118) (-26.5399, -3.8109) knots -0.013599 -0.013599 -0.013599 -0.013599 -0.010706 -0.010706 -0.007813 -0.007813 -0.003906 -0.003906 0 0 0 0
  arc A4 (-26.4478, -3.8961) -> (-26.3573, -4.4674) centre (0, 0) ccw
  spline S8 degree 3 poles (-26.4186, -4.5769) (-26.4096, -4.5733) (-26.4012, -4.5684) (-26.3861, -4.5564) (-26.3795, -4.5494) (-26.3665, -4.5308) (-26.3612, -4.5188) (-26.3555, -4.4934) (-26.3551, -4.4803) (-26.3573, -4.4674) knots -0.013599 -0.013599 -0.013599 -0.013599 -0.010706 -0.010706 -0.007813 -0.007813 -0.003906 -0.003906 0 0 0 0
  spline S9 degree 3 poles (-28.2737, -5.6363) (-27.9719, -5.4182) (-27.6537, -5.2098) (-27.0417, -4.8598) (-26.7296, -4.702) (-26.4186, -4.5769) knots -0.220678 -0.220678 -0.220678 -0.220678 -0.107909 -0.107909 -0.008028 -0.008028 -0.008028 -0.008028
  arc A5 (-28.2737, -5.6363) -> (-28.1218, -6.351) centre (0, 0) ccw
  spline S10 degree 3 poles (-25.9962, -6.5642) (-26.3312, -6.5765) (-26.6805, -6.5592) (-27.3819, -6.4884) (-27.7574, -6.4275) (-28.1218, -6.351) knots -0.210627 -0.210627 -0.210627 -0.210627 -0.111696 -0.111696 0 0 0 0
  spline S11 degree 3 poles (-25.8956, -6.6393) (-25.898, -6.6299) (-25.9018, -6.621) (-25.9117, -6.6045) (-25.9178, -6.5969) (-25.9345, -6.5816) (-25.9457, -6.5748) (-25.9702, -6.5658) (-25.9831, -6.5637) (-25.9962, -6.5642) knots -0.013599 -0.013599 -0.013599 -0.013599 -0.010706 -0.010706 -0.007813 -0.007813 -0.003906 -0.003906 0 0 0 0
  arc A6 (-25.8956, -6.6393) -> (-25.7459, -7.198) centre (0, 0) ccw
  spline S12 degree 3 poles (-25.7954, -7.3133) (-25.7869, -7.3088) (-25.7791, -7.3031) (-25.7653, -7.2896) (-25.7594, -7.2819) (-25.7485, -7.2621) (-25.7444, -7.2495) (-25.7414, -7.2237) (-25.7424, -7.2106) (-25.7459, -7.198) knots -0.013599 -0.013599 -0.013599 -0.013599 -0.010706 -0.010706 -0.007813 -0.007813 -0.003906 -0.003906 0 0 0 0
  spline S13 degree 3 poles (-27.5296, -8.5608) (-27.2523, -8.3124) (-26.9576, -8.0719) (-26.3856, -7.6598) (-26.0917, -7.4702) (-25.7954, -7.3133) knots -0.220678 -0.220678 -0.220678 -0.220678 -0.107909 -0.107909 -0.008028 -0.008028 -0.008028 -0.008028
  arc A7 (-27.5296, -8.5608) -> (-27.3039, -9.2557) centre (0, 0) ccw
  spline S14 degree 3 poles (-25.1676, -9.2456) (-25.4995, -9.2928) (-25.8487, -9.3122) (-26.5537, -9.315) (-26.9335, -9.2937) (-27.3039, -9.2557) knots -0.210627 -0.210627 -0.210627 -0.210627 -0.111696 -0.111696 0 0 0 0
  spline S15 degree 3 poles (-25.0598, -9.3097) (-25.0631, -9.3007) (-25.0678, -9.2922) (-25.0794, -9.2768) (-25.0863, -9.27) (-25.1045, -9.2565) (-25.1163, -9.2508) (-25.1416, -9.2444) (-25.1547, -9.2437) (-25.1676, -9.2456) knots -0.013599 -0.013599 -0.013599 -0.013599 -0.010706 -0.010706 -0.007813 -0.007813 -0.003906 -0.003906 0 0 0 0
  arc A8 (-25.0598, -9.3097) -> (-24.8525, -9.8498) centre (0, 0) ccw
  spline S16 degree 3 poles (-24.8897, -9.9696) (-24.8817, -9.9642) (-24.8745, -9.9577) (-24.8622, -9.9429) (-24.8572, -9.9346) (-24.8483, -9.9137) (-24.8456, -9.9008) (-24.8453, -9.8748) (-24.8477, -9.8619) (-24.8525, -9.8498) knots -0.013599 -0.013599 -0.013599 -0.013599 -0.010706 -0.010706 -0.007813 -0.007813 -0.003906 -0.003906 0 0 0 0
  spline S17 degree 3 poles (-26.484, -11.3915) (-26.2342, -11.1155) (-25.9662, -10.8455) (-25.4404, -10.3759) (-25.1679, -10.1566) (-24.8897, -9.9696) knots -0.220678 -0.220678 -0.220678 -0.220678 -0.107909 -0.107909 -0.008028 -0.008028 -0.008028 -0.008028
  arc A9 (-26.484, -11.3915) -> (-26.1868, -12.059) centre (0, 0) ccw
  spline S18 degree 3 poles (-24.0633, -11.8257) (-24.3884, -11.9073) (-24.7337, -11.9631) (-25.4345, -12.0396) (-25.8145, -12.0581) (-26.1868, -12.059) knots -0.210627 -0.210627 -0.210627 -0.210627 -0.111696 -0.111696 0 0 0 0
  spline S19 degree 3 poles (-23.9494, -11.8782) (-23.9537, -11.8696) (-23.9592, -11.8616) (-23.9723, -11.8475) (-23.9799, -11.8414) (-23.9994, -11.8299) (-24.0118, -11.8255) (-24.0376, -11.8218) (-24.0507, -11.8225) (-24.0633, -11.8257) knots -0.013599 -0.013599 -0.013599 -0.013599 -0.010706 -0.010706 -0.007813 -0.007813 -0.003906 -0.003906 0 0 0 0
  arc A10 (-23.9494, -11.8782) -> (-23.6868, -12.3936) centre (0, 0) ccw
  spline S20 degree 3 poles (-23.7112, -12.5167) (-23.7038, -12.5105) (-23.6974, -12.5033) (-23.6867, -12.4872) (-23.6826, -12.4784) (-23.6759, -12.4568) (-23.6746, -12.4437) (-23.677, -12.4178) (-23.6807, -12.4051) (-23.6868, -12.3936) knots -0.013599 -0.013599 -0.013599 -0.013599 -0.010706 -0.010706 -0.007813 -0.007813 -0.003906 -0.003906 0 0 0 0
  spline S21 degree 3 poles (-25.1482, -14.0975) (-24.9286, -13.7968) (-24.6903, -13.5003) (-24.2164, -12.9783) (-23.9684, -12.7317) (-23.7112, -12.5167) knots -0.220678 -0.220678 -0.220678 -0.220678 -0.107909 -0.107909 -0.008028 -0.008028 -0.008028 -0.008028
  arc A11 (-25.1482, -14.0975) -> (-24.7828, -14.7302) centre (0, 0) ccw
  spline S22 degree 3 poles (-22.6954, -14.2762) (-23.0102, -14.3914) (-23.3477, -14.4829) (-24.0367, -14.6323) (-24.4127, -14.6904) (-24.7828, -14.7302) knots -0.210627 -0.210627 -0.210627 -0.210627 -0.111696 -0.111696 0 0 0 0
  spline S23 degree 3 poles (-22.5766, -14.3165) (-22.5817, -14.3084) (-22.588, -14.301) (-22.6026, -14.2884) (-22.6107, -14.2831) (-22.6313, -14.2737) (-22.6441, -14.2707) (-22.6702, -14.2697) (-22.6831, -14.2717) (-22.6954, -14.2762) knots -0.013599 -0.013599 -0.013599 -0.013599 -0.010706 -0.010706 -0.007813 -0.007813 -0.003906 -0.003906 0 0 0 0
  arc A12 (-22.5766, -14.3165) -> (-22.2615, -14.8017) centre (0, 0) ccw
  spline S24 degree 3 poles (-22.273, -14.9266) (-22.2663, -14.9197) (-22.2606, -14.9118) (-22.2517, -14.8947) (-22.2485, -14.8856) (-22.2441, -14.8633) (-22.2442, -14.8502) (-22.2493, -14.8246) (-22.2543, -14.8125) (-22.2615, -14.8017) knots -0.013599 -0.013599 -0.013599 -0.013599 -0.010706 -0.010706 -0.007813 -0.007813 -0.003906 -0.003906 0 0 0 0
  spline S25 degree 3 poles (-23.5368, -16.6489) (-23.3499, -16.327) (-23.1439, -16.0071) (-22.7272, -15.4385) (-22.5063, -15.1674) (-22.273, -14.9266) knots -0.220678 -0.220678 -0.220678 -0.220678 -0.107909 -0.107909 -0.008028 -0.008028 -0.008028 -0.008028
  arc A13 (-23.5368, -16.6489) -> (-23.1074, -17.24) centre (0, 0) ccw
  spline S26 degree 3 poles (-21.0788, -16.5703) (-21.3798, -16.7177) (-21.7059, -16.8441) (-22.3755, -17.0646) (-22.7434, -17.1617) (-23.1074, -17.24) knots -0.210627 -0.210627 -0.210627 -0.210627 -0.111696 -0.111696 0 0 0 0
  spline S27 degree 3 poles (-20.9564, -16.598) (-20.9624, -16.5904) (-20.9694, -16.5838) (-20.9852, -16.5727) (-20.9939, -16.5683) (-21.0154, -16.5611) (-21.0284, -16.5594) (-21.0544, -16.5612) (-21.0671, -16.5645) (-21.0788, -16.5703) knots -0.013599 -0.013599 -0.013599 -0.013599 -0.010706 -0.010706 -0.007813 -0.007813 -0.003906 -0.003906 0 0 0 0
  arc A14 (-20.9564, -16.598) -> (-20.5924, -17.0475) centre (0, 0) ccw
  spline S28 degree 3 poles (-20.5907, -17.173) (-20.5848, -17.1654) (-20.5799, -17.157) (-20.5728, -17.1391) (-20.5706, -17.1296) (-20.5686, -17.1071) (-20.5701, -17.094) (-20.5778, -17.0691) (-20.5841, -17.0576) (-20.5924, -17.0475) knots -0.013599 -0.013599 -0.013599 -0.013599 -0.010706 -0.010706 -0.007813 -0.007813 -0.003906 -0.003906 0 0 0 0
  spline S29 degree 3 poles (-21.6676, -19.018) (-21.5153, -18.6782) (-21.3439, -18.3387) (-20.9889, -17.7295) (-20.7975, -17.4368) (-20.5907, -17.173) knots -0.220678 -0.220678 -0.220678 -0.220678 -0.107909 -0.107909 -0.008028 -0.008028 -0.008028 -0.008028
  arc A15 (-21.6676, -19.018) -> (-21.1787, -19.561) centre (0, 0) ccw
  spline S30 degree 3 poles (-19.2312, -18.6828) (-19.5152, -18.861) (-19.8263, -19.0207) (-20.4692, -19.31) (-20.8249, -19.445) (-21.1787, -19.561) knots -0.210627 -0.210627 -0.210627 -0.210627 -0.111696 -0.111696 0 0 0 0
  spline S31 degree 3 poles (-19.1066, -18.6976) (-19.1134, -18.6907) (-19.1211, -18.6848) (-19.1379, -18.6755) (-19.147, -18.672) (-19.1691, -18.6671) (-19.1823, -18.6668) (-19.2079, -18.6712) (-19.2202, -18.6759) (-19.2312, -18.6828) knots -0.013599 -0.013599 -0.013599 -0.013599 -0.010706 -0.010706 -0.007813 -0.007813 -0.003906 -0.003906 0 0 0 0
  arc A16 (-19.1066, -18.6976) -> (-18.6976, -19.1066) centre (0, 0) ccw
  spline S32 degree 3 poles (-18.6828, -19.2312) (-18.6777, -19.2231) (-18.6738, -19.2142) (-18.6686, -19.1956) (-18.6674, -19.186) (-18.6678, -19.1633) (-18.6706, -19.1505) (-18.6809, -19.1266) (-18.6883, -19.1157) (-18.6976, -19.1066) knots -0.013599 -0.013599 -0.013599 -0.013599 -0.010706 -0.010706 -0.007813 -0.007813 -0.003906 -0.003906 0 0 0 0
  spline S33 degree 3 poles (-19.561, -21.1787) (-19.445, -20.8249) (-19.31, -20.4692) (-19.0207, -19.8263) (-18.861, -19.5152) (-18.6828, -19.2312) knots -0.220678 -0.220678 -0.220678 -0.220678 -0.107909 -0.107909 -0.008028 -0.008028 -0.008028 -0.008028
  arc A17 (-19.561, -21.1787) -> (-19.018, -21.6676) centre (0, 0) ccw
  spline S34 degree 3 poles (-17.173, -20.5907) (-17.4368, -20.7975) (-17.7295, -20.9889) (-18.3387, -21.3439) (-18.6782, -21.5153) (-19.018, -21.6676) knots -0.210627 -0.210627 -0.210627 -0.210627 -0.111696 -0.111696 0 0 0 0
  spline S35 degree 3 poles (-17.0475, -20.5924) (-17.055, -20.5862) (-17.0632, -20.5812) (-17.081, -20.5736) (-17.0904, -20.5711) (-17.1129, -20.5686) (-17.126, -20.5696) (-17.151, -20.5767) (-17.1628, -20.5827) (-17.173, -20.5907) knots -0.013599 -0.013599 -0.013599 -0.013599 -0.010706 -0.010706 -0.007813 -0.007813 -0.003906 -0.003906 0 0 0 0
  arc A18 (-17.0475, -20.5924) -> (-16.598, -20.9564) centre (0, 0) ccw
  spline S36 degree 3 poles (-16.5703, -21.0788) (-16.566, -21.0701) (-16.5631, -21.0609) (-16.5599, -21.0419) (-16.5597, -21.0322) (-16.5624, -21.0097) (-16.5665, -20.9972) (-16.5793, -20.9745) (-16.5878, -20.9645) (-16.598, -20.9564) knots -0.013599 -0.013599 -0.013599 -0.013599 -0.010706 -0.010706 -0.007813 -0.007813 -0.003906 -0.003906 0 0 0 0
  spline S37 degree 3 poles (-17.24, -23.1074) (-17.1617, -22.7434) (-17.0646, -22.3755) (-16.8441, -21.7059) (-16.7177, -21.3798) (-16.5703, -21.0788) knots -0.220678 -0.220678 -0.220678 -0.220678 -0.107909 -0.107909 -0.008028 -0.008028 -0.008028 -0.008028
  arc A19 (-17.24, -23.1074) -> (-16.6489, -23.5368) centre (0, 0) ccw
  spline S38 degree 3 poles (-14.9266, -22.273) (-15.1674, -22.5063) (-15.4385, -22.7272) (-16.0071, -23.1439) (-16.327, -23.3499) (-16.6489, -23.5368) knots -0.210627 -0.210627 -0.210627 -0.210627 -0.111696 -0.111696 0 0 0 0
  spline S39 degree 3 poles (-14.8017, -22.2615) (-14.8097, -22.2562) (-14.8184, -22.252) (-14.8369, -22.2464) (-14.8465, -22.2449) (-14.8691, -22.2447) (-14.882, -22.2471) (-14.9062, -22.2568) (-14.9173, -22.2639) (-14.9266, -22.273) knots -0.013599 -0.013599 -0.013599 -0.013599 -0.010706 -0.010706 -0.007813 -0.007813 -0.003906 -0.003906 0 0 0 0
  arc A20 (-14.8017, -22.2615) -> (-14.3165, -22.5766) centre (0, 0) ccw
  spline S40 degree 3 poles (-14.2762, -22.6954) (-14.2729, -22.6863) (-14.2709, -22.6768) (-14.2697, -22.6576) (-14.2705, -22.6479) (-14.2756, -22.6258) (-14.2809, -22.6138) (-14.296, -22.5926) (-14.3055, -22.5835) (-14.3165, -22.5766) knots -0.013599 -0.013599 -0.013599 -0.013599 -0.010706 -0.010706 -0.007813 -0.007813 -0.003906 -0.003906 0 0 0 0
  spline S41 degree 3 poles (-14.7302, -24.7828) (-14.6904, -24.4127) (-14.6323, -24.0367) (-14.4829, -23.3477) (-14.3914, -23.0102) (-14.2762, -22.6954) knots -0.220678 -0.220678 -0.220678 -0.220678 -0.107909 -0.107909 -0.008028 -0.008028 -0.008028 -0.008028
  arc A21 (-14.7302, -24.7828) -> (-14.0975, -25.1482) centre (0, 0) ccw
  spline S42 degree 3 poles (-12.5167, -23.7112) (-12.7317, -23.9684) (-12.9783, -24.2164) (-13.5003, -24.6903) (-13.7968, -24.9286) (-14.0975, -25.1482) knots -0.210627 -0.210627 -0.210627 -0.210627 -0.111696 -0.111696 0 0 0 0
  spline S43 degree 3 poles (-12.3936, -23.6868) (-12.4022, -23.6823) (-12.4113, -23.6791) (-12.4302, -23.6754) (-12.4399, -23.6749) (-12.4625, -23.6771) (-12.4751, -23.6808) (-12.4981, -23.693) (-12.5083, -23.7012) (-12.5167, -23.7112) knots -0.013599 -0.013599 -0.013599 -0.013599 -0.010706 -0.010706 -0.007813 -0.007813 -0.003906 -0.003906 0 0 0 0
  arc A22 (-12.3936, -23.6868) -> (-11.8782, -23.9494) centre (0, 0) ccw
  spline S44 degree 3 poles (-11.8257, -24.0633) (-11.8233, -24.054) (-11.8223, -24.0443) (-11.8231, -24.025) (-11.8249, -24.0155) (-11.8323, -23.9941) (-11.8389, -23.9827) (-11.8561, -23.9632) (-11.8665, -23.9552) (-11.8782, -23.9494) knots -0.013599 -0.013599 -0.013599 -0.013599 -0.010706 -0.010706 -0.007813 -0.007813 -0.003906 -0.003906 0 0 0 0
  spline S45 degree 3 poles (-12.059, -26.1868) (-12.0581, -25.8145) (-12.0396, -25.4345) (-11.9631, -24.7337) (-11.9073, -24.3884) (-11.8257, -24.0633) knots -0.220678 -0.220678 -0.220678 -0.220678 -0.107909 -0.107909 -0.008028 -0.008028 -0.008028 -0.008028
  arc A23 (-12.059, -26.1868) -> (-11.3915, -26.484) centre (0, 0) ccw
  spline S46 degree 3 poles (-9.9696, -24.8897) (-10.1566, -25.1679) (-10.3759, -25.4404) (-10.8455, -25.9662) (-11.1155, -26.2342) (-11.3915, -26.484) knots -0.210627 -0.210627 -0.210627 -0.210627 -0.111696 -0.111696 0 0 0 0
  spline S47 degree 3 poles (-9.8498, -24.8525) (-9.8587, -24.8489) (-9.8682, -24.8467) (-9.8874, -24.845) (-9.8971, -24.8455) (-9.9193, -24.85) (-9.9314, -24.8551) (-9.9531, -24.8696) (-9.9624, -24.8789) (-9.9696, -24.8897) knots -0.013599 -0.013599 -0.013599 -0.013599 -0.010706 -0.010706 -0.007813 -0.007813 -0.003906 -0.003906 0 0 0 0
  arc A24 (-9.8498, -24.8525) -> (-9.3097, -25.0598) centre (0, 0) ccw
  spline S48 degree 3 poles (-9.2456, -25.1676) (-9.2442, -25.1581) (-9.2442, -25.1484) (-9.2471, -25.1293) (-9.2499, -25.12) (-9.2594, -25.0995) (-9.2672, -25.0888) (-9.2863, -25.0712) (-9.2975, -25.0643) (-9.3097, -25.0598) knots -0.013599 -0.013599 -0.013599 -0.013599 -0.010706 -0.010706 -0.007813 -0.007813 -0.003906 -0.003906 0 0 0 0
  spline S49 degree 3 poles (-9.2557, -27.3039) (-9.2937, -26.9335) (-9.315, -26.5537) (-9.3122, -25.8487) (-9.2928, -25.4995) (-9.2456, -25.1676) knots -0.220678 -0.220678 -0.220678 -0.220678 -0.107909 -0.107909 -0.008028 -0.008028 -0.008028 -0.008028
  arc A25 (-9.2557, -27.3039) -> (-8.5608, -27.5296) centre (0, 0) ccw
  spline S50 degree 3 poles (-7.3133, -25.7954) (-7.4702, -26.0917) (-7.6598, -26.3856) (-8.0719, -26.9576) (-8.3124, -27.2523) (-8.5608, -27.5296) knots -0.210627 -0.210627 -0.210627 -0.210627 -0.111696 -0.111696 0 0 0 0
  spline S51 degree 3 poles (-7.198, -25.7459) (-7.2073, -25.7433) (-7.2169, -25.7421) (-7.2362, -25.7424) (-7.2458, -25.7439) (-7.2674, -25.7508) (-7.2789, -25.757) (-7.2989, -25.7737) (-7.3072, -25.7839) (-7.3133, -25.7954) knots -0.013599 -0.013599 -0.013599 -0.013599 -0.010706 -0.010706 -0.007813 -0.007813 -0.003906 -0.003906 0 0 0 0
  arc A26 (-7.198, -25.7459) -> (-6.6393, -25.8956) centre (0, 0) ccw
  spline S52 degree 3 poles (-6.5642, -25.9962) (-6.5638, -25.9865) (-6.5649, -25.9769) (-6.5697, -25.9582) (-6.5734, -25.9493) (-6.5851, -25.9298) (-6.5939, -25.9201) (-6.6148, -25.9045) (-6.6267, -25.8989) (-6.6393, -25.8956) knots -0.013599 -0.013599 -0.013599 -0.013599 -0.010706 -0.010706 -0.007813 -0.007813 -0.003906 -0.003906 0 0 0 0
  spline S53 degree 3 poles (-6.351, -28.1218) (-6.4275, -27.7574) (-6.4884, -27.3819) (-6.5592, -26.6805) (-6.5765, -26.3312) (-6.5642, -25.9962) knots -0.220678 -0.220678 -0.220678 -0.220678 -0.107909 -0.107909 -0.008028 -0.008028 -0.008028 -0.008028
  arc A27 (-6.351, -28.1218) -> (-5.6363, -28.2737) centre (0, 0) ccw
  spline S54 degree 3 poles (-4.5769, -26.4186) (-4.702, -26.7296) (-4.8598, -27.0417) (-5.2098, -27.6537) (-5.4182, -27.9719) (-5.6363, -28.2737) knots -0.210627 -0.210627 -0.210627 -0.210627 -0.111696 -0.111696 0 0 0 0
  spline S55 degree 3 poles (-4.4674, -26.3573) (-4.4769, -26.3557) (-4.4866, -26.3554) (-4.5058, -26.3578) (-4.5151, -26.3603) (-4.5359, -26.3693) (-4.5467, -26.3768) (-4.5649, -26.3955) (-4.572, -26.4065) (-4.5769, -26.4186) knots -0.013599 -0.013599 -0.013599 -0.013599 -0.010706 -0.010706 -0.007813 -0.007813 -0.003906 -0.003906 0 0 0 0
  arc A28 (-4.4674, -26.3573) -> (-3.8961, -26.4478) centre (0, 0) ccw
  spline S56 degree 3 poles (-3.8109, -26.5399) (-3.8115, -26.5303) (-3.8136, -26.5208) (-3.8203, -26.5027) (-3.825, -26.4942) (-3.8386, -26.4761) (-3.8484, -26.4674) (-3.8708, -26.4541) (-3.8832, -26.4497) (-3.8961, -26.4478) knots -0.013599 -0.013599 -0.013599 -0.013599 -0.010706 -0.010706 -0.007813 -0.007813 -0.003906 -0.003906 0 0 0 0
  spline S57 degree 3 poles (-3.3766, -28.6316) (-3.4908, -28.2772) (-3.5906, -27.9101) (-3.7344, -27.2199) (-3.7881, -26.8744) (-3.8109, -26.5399) knots -0.220678 -0.220678 -0.220678 -0.220678 -0.107909 -0.107909 -0.008028 -0.008028 -0.008028 -0.008028
  arc A29 (-3.3766, -28.6316) -> (-2.65, -28.708) centre (0, 0) ccw
  spline S58 degree 3 poles (-1.7903, -26.7523) (-1.8822, -27.0747) (-2.0065, -27.4015) (-2.2907, -28.0467) (-2.4646, -28.385) (-2.65, -28.708) knots -0.210627 -0.210627 -0.210627 -0.210627 -0.111696 -0.111696 0 0 0 0
  spline S59 degree 3 poles (-1.6879, -26.6799) (-1.6975, -26.6793) (-1.7071, -26.68) (-1.7259, -26.6844) (-1.735, -26.6879) (-1.7547, -26.699) (-1.7647, -26.7076) (-1.7808, -26.728) (-1.7868, -26.7397) (-1.7903, -26.7523) knots -0.013599 -0.013599 -0.013599 -0.013599 -0.010706 -0.010706 -0.007813 -0.007813 -0.003906 -0.003906 0 0 0 0
  arc A30 (-1.6879, -26.6799) -> (-1.1102, -26.7101) centre (0, 0) ccw
  spline S60 degree 3 poles (-1.0158, -26.7929) (-1.0175, -26.7834) (-1.0205, -26.7741) (-1.0291, -26.7569) (-1.0346, -26.7489) (-1.0501, -26.7323) (-1.0607, -26.7246) (-1.0844, -26.7138) (-1.0972, -26.7107) (-1.1102, -26.7101) knots -0.013599 -0.013599 -0.013599 -0.013599 -0.010706 -0.010706 -0.007813 -0.007813 -0.003906 -0.003906 0 0 0 0
  spline S61 degree 3 poles (-0.3653, -28.8277) (-0.5159, -28.4872) (-0.6536, -28.1325) (-0.8687, -27.4612) (-0.9582, -27.1231) (-1.0158, -26.7929) knots -0.220678 -0.220678 -0.220678 -0.220678 -0.107909 -0.107909 -0.008028 -0.008028 -0.008028 -0.008028
  arc A31 (-0.3653, -28.8277) -> (0.3653, -28.8277) centre (0, 0) ccw